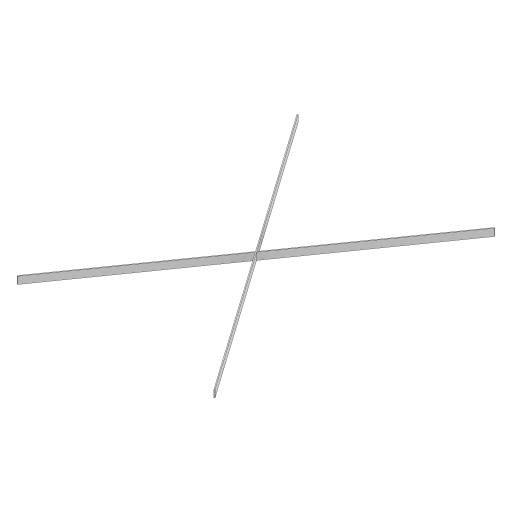
# Autodesk Inventor part: PLETINA DE INERCIA
Saved by Autodesk Inventor 2024 (Build 280153000, 153)
## iProperties
Created: 2024-06-13
Part Number: PLETINA DE INERCIA
Material: Generic
Document SubType Name: Modeling
Designer: Jhuliams
Density: 1 g/cm^3
Appearance: Default
Author: Jhuliams
Autodesk Inventor part; units mm, degrees
ref_plane "YZ Plane" through (0, 0, 0) normal (1, 0, 0) x (0, 1, 0)
ref_plane "XZ Plane" through (0, 0, 0) normal (0, 1, 0) x (-1, 0, 0)
ref_plane "XY Plane" through (0, 0, 0) normal (0, 0, 1) x (1, 0, 0)
sketch "Sketch3" plane through (0, 0, 0) normal (0, 1, 0) x (-1, 0, 0)
  line L0 (344.5, 490) -> (-344.5, 490)
  line L1 (-344.5, 490) -> (-344.5, -490)
  line L2 (-344.5, -490) -> (344.5, -490)
  line L3 (344.5, -490) -> (344.5, 490)
  line L4 (344.5, 490) -> (-344.5, -490) construction
  line L5 (-344.5, 490) -> (344.5, -490) construction
  line L6 (344.5, 490) -> (-344.5, -490)
  line L7 (344.5, -490) -> (-344.5, 490)
  line L8 (345.7271, 489.1373) -> (-343.2729, -490.8627)
  line L9 (343.2729, 490.8627) -> (-345.7271, -489.1373)
  line L10 (-343.2729, 490.8627) -> (345.7271, -489.1373)
  line L11 (343.2729, -490.8627) -> (-345.7271, 489.1373)
  point P0 (0, 0)
  point P1 (0, -2.6081)
  point P2 (342.6664, -490)
  point P3 (344.5, -487.3919)
  point P4 (1.8336, 0)
  point P5 (344.5, 487.3919)
  point P6 (342.6664, 490)
  point P7 (0, 2.6081)
  point P8 (-342.6664, 490)
  point P9 (-344.5, 487.3919)
  point P10 (-1.8336, 0)
  point P11 (-344.5, -487.3919)
  point P12 (-342.6664, -490)
  dimension "d13" = 689
  dimension "d14" = 980
  dimension "d15" = 1.5
  dimension "d16" = 1.5
  dimension "d17" = 1.5
  dimension "d18" = 1.5
  constraints: 24 end point, 7 equal length, 2 midpoint, 1 horizontal, 1 perpendicular
  measures "d13" distance of L2.end L1.end
  measures "d14" distance of L1.end L0.end
  measures "d15" distance between parallel lines of L4 L8
  measures "d16" distance between parallel lines of L4 L9
  measures "d17" distance between parallel lines of L5 L10
  measures "d18" distance between parallel lines of L7 L11
extrude "Extrusion3" add sketch "Sketch3" along normal blind 25 contours L6 L10 L9 L0 | L3 L8 L10 L6 | L10 L8 L7 L6 | L6 L7 L9 L10 | L10 L9 L7 L0 | L3 L7 L8 L10 | L7 L8 L11 L6 | L6 L11 L9 L7 | L7 L9 L11 L1 | L2 L11 L8 L7 | L11 L8 L2 L6 | L6 L1 L9 L11
body "Solid3"
